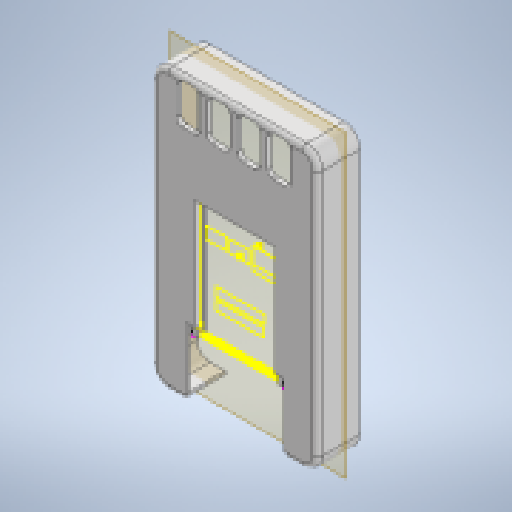
# Autodesk Inventor part: Top Housing
Saved by Autodesk Inventor 2023 (Build 270158000, 158)
## iProperties
Created: 2024-03-21
Part Number: Top Housing
Material: Generic
Document SubType Name: Modeling
Designer: Pobe Tran
Density: 1 g/cm^3
Appearance: Default
Author: Pobe Tran
Autodesk Inventor part; units mm, degrees
sketch "Sketch1" plane through (0, 0, 0) normal (0, 0, 1) x (1, 0, 0)
  point P0 (0, 0)
ref_plane "Work Plane1" through (48, 84.1076, 7.5) normal (0, 0, 1) x (1, 0, 0)
ref_plane "Work Plane2" through (-0.3396, -5.2087, 0) normal (0, 0, 1) x (1, 0, 0)
sketch "Sketch7" plane through (-0.3396, -5.2087, 0) normal (0, 0, 1) x (1, 0, 0)
  line L0 (50.1982, -77.6837) -> (50.1982, 77.6837) projected
  arc A0 (42.1982, -85.6837) -> (50.1982, -77.6837) centre (42.1982, -77.6837) ccw projected
  line L1 (-42.1982, -85.6837) -> (42.1982, -85.6837) projected
  line L2 (42.1982, -87.6837) -> (-42.1982, -87.6837) projected
  arc A1 (42.1982, -87.6837) -> (52.1982, -77.6837) centre (42.1982, -77.6837) ccw projected
  line L3 (52.1982, 77.6837) -> (52.1982, -77.6837) projected
  arc A2 (52.1982, 77.6837) -> (42.1982, 87.6837) centre (42.1982, 77.6837) ccw projected
  arc A3 (50.1982, 77.6837) -> (42.1982, 85.6837) centre (42.1982, 77.6837) ccw projected
  line L4 (-42.1982, 87.6837) -> (42.1982, 87.6837) projected
  line L5 (42.1982, 85.6837) -> (-42.1982, 85.6837) projected
  arc A4 (-42.1982, 87.6837) -> (-52.1982, 77.6837) centre (-42.1982, 77.6837) ccw projected
  arc A5 (-42.1982, 85.6837) -> (-50.1982, 77.6837) centre (-42.1982, 77.6837) ccw projected
  line L6 (-50.1982, 77.6837) -> (-50.1982, -77.6837) projected
  line L7 (-52.1982, -77.6837) -> (-52.1982, 77.6837) projected
  arc A6 (-52.1982, -77.6837) -> (-42.1982, -87.6837) centre (-42.1982, -77.6837) ccw projected
  arc A7 (-50.1982, -77.6837) -> (-42.1982, -85.6837) centre (-42.1982, -77.6837) ccw projected
  point P0 (0.3396, 5.2087)
extrude "Extrusion5" add sketch "Sketch7" along normal blind 11.5 and the other way blind 12
sketch "Sketch8" plane through (-0.3396, -5.2087, 11.5) normal (0, 0, 1) x (1, 0, 0)
  line L0 (52.1982, -77.6837) -> (52.1982, 77.6837) projected
  arc A0 (42.1982, -87.6837) -> (52.1982, -77.6837) centre (42.1982, -77.6837) ccw projected
  line L1 (-42.1982, -87.6837) -> (42.1982, -87.6837) projected
  arc A1 (-52.1982, -77.6837) -> (-42.1982, -87.6837) centre (-42.1982, -77.6837) ccw projected
  line L2 (-52.1982, 77.6837) -> (-52.1982, -77.6837) projected
  arc A2 (-42.1982, 87.6837) -> (-52.1982, 77.6837) centre (-42.1982, 77.6837) ccw projected
  line L3 (42.1982, 87.6837) -> (-42.1982, 87.6837) projected
  arc A3 (52.1982, 77.6837) -> (42.1982, 87.6837) centre (42.1982, 77.6837) ccw projected
  point P0 (0.3396, 5.2087)
extrude "Extrusion6" add sketch "Sketch8" along normal blind 3
sketch "Sketch9" plane through (-0.3396, -5.2087, 14.5) normal (0, 0, 1) x (1, 0, 0)
  arc A0 (31.6451, 60.9262) -> (34.8201, 64.1012) centre (31.6451, 64.1012) ccw projected
  line L0 (34.8201, 64.1012) -> (34.8201, 81.8812) projected
  arc A1 (34.8201, 81.8812) -> (31.6451, 85.0562) centre (31.6451, 81.8812) ccw projected
  line L1 (31.6451, 85.0562) -> (24.0251, 85.0562) projected
  arc A2 (24.0251, 85.0562) -> (20.8501, 81.8812) centre (24.0251, 81.8812) ccw projected
  line L2 (20.8501, 81.8812) -> (20.8501, 64.1012) projected
  arc A3 (20.8501, 64.1012) -> (24.0251, 60.9262) centre (24.0251, 64.1012) ccw projected
  line L3 (24.0251, 60.9262) -> (31.6451, 60.9262) projected
  arc A4 (12.5951, 60.9262) -> (15.7701, 64.1012) centre (12.5951, 64.1012) ccw projected
  line L4 (15.7701, 64.1012) -> (15.7701, 81.8812) projected
  arc A5 (15.7701, 81.8812) -> (12.5951, 85.0562) centre (12.5951, 81.8812) ccw projected
  line L5 (12.5951, 85.0562) -> (4.9751, 85.0562) projected
  arc A6 (4.9751, 85.0562) -> (1.8001, 81.8812) centre (4.9751, 81.8812) ccw projected
  line L6 (1.8001, 81.8812) -> (1.8001, 64.1012) projected
  arc A7 (1.8001, 64.1012) -> (4.9751, 60.9262) centre (4.9751, 64.1012) ccw projected
  line L7 (4.9751, 60.9262) -> (12.5951, 60.9262) projected
  arc A8 (-6.4549, 60.9262) -> (-3.2799, 64.1012) centre (-6.4549, 64.1012) ccw projected
  line L8 (-3.2799, 64.1012) -> (-3.2799, 81.8812) projected
  arc A9 (-3.2799, 81.8812) -> (-6.4549, 85.0562) centre (-6.4549, 81.8812) ccw projected
  line L9 (-6.4549, 85.0562) -> (-14.0749, 85.0562) projected
  arc A10 (-14.0749, 85.0562) -> (-17.2499, 81.8812) centre (-14.0749, 81.8812) ccw projected
  line L10 (-17.2499, 81.8812) -> (-17.2499, 64.1012) projected
  arc A11 (-17.2499, 64.1012) -> (-14.0749, 60.9262) centre (-14.0749, 64.1012) ccw projected
  line L11 (-14.0749, 60.9262) -> (-6.4549, 60.9262) projected
  arc A12 (-25.5049, 60.9262) -> (-22.3299, 64.1012) centre (-25.5049, 64.1012) ccw projected
  line L12 (-22.3299, 64.1012) -> (-22.3299, 81.8812) projected
  arc A13 (-22.3299, 81.8812) -> (-25.5049, 85.0562) centre (-25.5049, 81.8812) ccw projected
  line L13 (-25.5049, 85.0562) -> (-33.1249, 85.0562) projected
  arc A14 (-33.1249, 85.0562) -> (-36.2999, 81.8812) centre (-33.1249, 81.8812) ccw projected
  line L14 (-36.2999, 81.8812) -> (-36.2999, 64.1012) projected
  arc A15 (-36.2999, 64.1012) -> (-33.1249, 60.9262) centre (-33.1249, 64.1012) ccw projected
  line L15 (-33.1249, 60.9262) -> (-25.5049, 60.9262) projected
  arc A16 (31.6451, 60.4262) -> (35.3201, 64.1012) centre (31.6451, 64.1012) ccw
  line L16 (35.3201, 64.1012) -> (35.3201, 81.8812)
  arc A17 (35.3201, 81.8812) -> (31.6451, 85.5562) centre (31.6451, 81.8812) ccw
  line L17 (31.6451, 85.5562) -> (24.0251, 85.5562)
  arc A18 (24.0251, 85.5562) -> (20.3501, 81.8812) centre (24.0251, 81.8812) ccw
  line L18 (20.3501, 81.8812) -> (20.3501, 64.1012)
  arc A19 (20.3501, 64.1012) -> (24.0251, 60.4262) centre (24.0251, 64.1012) ccw
  line L19 (24.0251, 60.4262) -> (31.6451, 60.4262)
  line L20 (16.2701, 81.8812) -> (16.2701, 64.1012)
  arc A20 (12.5951, 60.4262) -> (16.2701, 64.1012) centre (12.5951, 64.1012) ccw
  line L21 (12.5951, 60.4262) -> (4.9751, 60.4262)
  arc A21 (1.3001, 64.1012) -> (4.9751, 60.4262) centre (4.9751, 64.1012) ccw
  line L22 (1.3001, 64.1012) -> (1.3001, 81.8812)
  arc A22 (4.9751, 85.5562) -> (1.3001, 81.8812) centre (4.9751, 81.8812) ccw
  line L23 (4.9751, 85.5562) -> (12.5951, 85.5562)
  arc A23 (16.2701, 81.8812) -> (12.5951, 85.5562) centre (12.5951, 81.8812) ccw
  arc A24 (-6.4549, 60.4262) -> (-2.7799, 64.1012) centre (-6.4549, 64.1012) ccw
  line L24 (-2.7799, 64.1012) -> (-2.7799, 81.8812)
  arc A25 (-2.7799, 81.8812) -> (-6.4549, 85.5562) centre (-6.4549, 81.8812) ccw
  line L25 (-6.4549, 85.5562) -> (-14.0749, 85.5562)
  arc A26 (-14.0749, 85.5562) -> (-17.7499, 81.8812) centre (-14.0749, 81.8812) ccw
  line L26 (-17.7499, 81.8812) -> (-17.7499, 64.1012)
  arc A27 (-17.7499, 64.1012) -> (-14.0749, 60.4262) centre (-14.0749, 64.1012) ccw
  line L27 (-14.0749, 60.4262) -> (-6.4549, 60.4262)
  arc A28 (-25.5049, 60.4262) -> (-21.8299, 64.1012) centre (-25.5049, 64.1012) ccw
  line L28 (-25.5049, 60.4262) -> (-33.1249, 60.4262)
  arc A29 (-36.7999, 64.1012) -> (-33.1249, 60.4262) centre (-33.1249, 64.1012) ccw
  line L29 (-36.7999, 64.1012) -> (-36.7999, 81.8812)
  arc A30 (-33.1249, 85.5562) -> (-36.7999, 81.8812) centre (-33.1249, 81.8812) ccw
  line L30 (-33.1249, 85.5562) -> (-25.5049, 85.5562)
  arc A31 (-21.8299, 81.8812) -> (-25.5049, 85.5562) centre (-25.5049, 81.8812) ccw
  line L31 (-21.8299, 81.8812) -> (-21.8299, 64.1012)
  point P0 (0.3396, 5.2087)
  dimension "d28" = 0.5
  dimension "d29" = 0.5
  dimension "d30" = 0.5
  dimension "d31" = 0.5
  constraints: 32 end point, 32 point on circle, 16 centre point, 28 other
  measures "d28" distance between parallel lines of L3 L19
  measures "d29" distance between parallel lines of L4 L20
  measures "d30" distance between parallel lines of L11 L27
  measures "d31" radial gap between concentric circles of A12 A28
extrude "Extrusion7" cut sketch "Sketch9" against normal blind 3 contours L3 A3 L2 A2 L1 A1 L0 A0 | L7 A7 L6 A6 L5 A5 L4 A4 | L11 A11 L10 A10 L9 A9 L8 A8 | L15 A15 L14 A14 L13 A13 L12 A12 | L19 A19 L18 A18 L17 A17 L16 A16 | L20 A20 L21 A21 L22 A22 L23 A23 | L27 A27 L26 A26 L25 A25 L24 A24 | L28 A29 L29 A30 L30 A31 L31 A28
sketch "Sketch10" plane through (-0.3396, -5.2087, 14.5) normal (0, 0, 1) x (1, 0, 0)
  line L0 (25.0411, 23.7903) -> (-24.5651, 23.7903) projected
  line L1 (-24.5651, 23.7903) -> (-24.5651, -45.0437) projected
  line L2 (-24.5651, -45.0437) -> (25.0411, -45.0437) projected
  line L3 (25.0411, -45.0437) -> (25.0411, 23.7903) projected
  line L4 (-28.4005, 30.4451) -> (28.6225, 30.4451) projected
  line L5 (28.6225, -51.2159) -> (-28.4005, -51.2159) projected
  line L6 (-25.2255, -45.5009) -> (-25.2255, 24.7301) projected
  line L7 (25.5411, 24.2903) -> (-25.0651, 24.2903)
  line L8 (-25.0651, 24.2903) -> (-25.0651, -45.5437)
  line L9 (-25.0651, -45.5437) -> (25.5411, -45.5437)
  line L10 (25.5411, -45.5437) -> (25.5411, 24.2903)
  dimension "d34" = 0.5
  constraints: 8 end point, 3 other
  measures "d34" distance between parallel lines of L3 L10
extrude "Extrusion8" cut sketch "Sketch10" against normal blind 3 contours L3 L2 L1 L0 | L10 L9 L8 L7
fillet "Fillet1" radius 3.175 8 edges at (48.9297, 79.546, 14.5) (-0.3396, 82.475, 14.5) (-49.609, 79.546, 14.5) (-52.5379, -5.2087, 14.5) (-49.609, -89.9635, 14.5) (-0.3396, -92.8924, 14.5) (48.9297, -89.9635, 14.5) (51.8586, -5.2087, 14.5)
sketch "Sketch15" plane through (-0.3396, -5.2087, 11.5) normal (0, 0, -1) x (-1, 0, 0)
  line L0 (-28.6225, -51.2159) -> (28.4005, -51.2159) projected
  arc A0 (28.4005, -51.2159) -> (28.4005, -46.0089) centre (28.4005, -48.6124) ccw projected
  line L1 (28.4005, -46.0089) -> (25.7335, -46.0089) projected
  arc A1 (25.2255, -45.5009) -> (25.7335, -46.0089) centre (25.7335, -45.5009) ccw projected
  line L2 (25.2255, -45.5009) -> (25.2255, 24.7301) projected
  arc A2 (25.7335, 25.2381) -> (25.2255, 24.7301) centre (25.7335, 24.7301) ccw projected
  line L3 (25.7335, 25.2381) -> (28.4005, 25.2381) projected
  arc A3 (28.4005, 25.2381) -> (28.4005, 30.4451) centre (28.4005, 27.8416) ccw projected
  line L4 (28.4005, 30.4451) -> (-28.6225, 30.4451) projected
  arc A4 (-28.6225, 30.4451) -> (-28.6225, 25.2381) centre (-28.6225, 27.8416) ccw projected
  line L5 (-28.6225, 25.2381) -> (-25.9555, 25.2381) projected
  arc A5 (-25.4475, 24.7301) -> (-25.9555, 25.2381) centre (-25.9555, 24.7301) ccw projected
  line L6 (-25.4475, 24.7301) -> (-25.4475, -45.5009) projected
  arc A6 (-25.9555, -46.0089) -> (-25.4475, -45.5009) centre (-25.9555, -45.5009) ccw projected
  line L7 (-25.9555, -46.0089) -> (-28.6225, -46.0089) projected
  arc A7 (-28.6225, -46.0089) -> (-28.6225, -51.2159) centre (-28.6225, -48.6124) ccw projected
  circle A8 centre (-18.6861, 27.9216) radius 0.9995 projected
  circle A9 centre (-16.1861, 27.9216) radius 0.9995 projected
  circle A10 centre (-13.6861, 27.9216) radius 0.9995 projected
  circle A11 centre (-11.1861, 27.9216) radius 0.9995 projected
  circle A12 centre (-8.6861, 27.9216) radius 0.9995 projected
  circle A13 centre (-6.1861, 27.9216) radius 0.9995 projected
  circle A14 centre (-3.6861, 27.9216) radius 0.9995 projected
  circle A15 centre (-1.1861, 27.9216) radius 0.9995 projected
  circle A16 centre (1.3139, 27.9216) radius 0.9995 projected
  circle A17 centre (3.8139, 27.9216) radius 0.9995 projected
  circle A18 centre (6.3139, 27.9216) radius 0.9995 projected
  circle A19 centre (8.8139, 27.9216) radius 0.9995 projected
  circle A20 centre (11.3139, 27.9216) radius 0.9995 projected
  circle A21 centre (13.8139, 27.9216) radius 0.9995 projected
  circle A22 centre (16.3139, 27.9216) radius 0.9995 projected
  circle A23 centre (18.8139, 27.9216) radius 0.9995 projected
  circle A24 centre (21.3139, 27.9216) radius 0.9995 projected
  line L8 (24.8139, -49.6924) -> (24.8139, -47.6924) projected
  line L9 (22.8139, -49.6924) -> (24.8139, -49.6924) projected
  line L10 (22.8139, -47.6924) -> (22.8139, -49.6924) projected
  line L11 (24.8139, -47.6924) -> (22.8139, -47.6924) projected
  line L12 (21.5552, 3.8513) -> (21.5552, 11.3443) projected
  line L13 (8.6012, 3.8513) -> (21.5552, 3.8513) projected
  line L14 (8.6012, 11.3443) -> (8.6012, 3.8513) projected
  line L15 (21.5552, 11.3443) -> (8.6012, 11.3443) projected
  line L16 (6.5692, 3.8513) -> (6.5692, 11.3443) projected
  line L17 (-6.3848, 3.8513) -> (6.5692, 3.8513) projected
  line L18 (-6.3848, 11.3443) -> (-6.3848, 3.8513) projected
  line L19 (6.5692, 11.3443) -> (-6.3848, 11.3443) projected
  line L20 (15.3703, -24.4189) -> (15.3703, -18.9325) projected
  line L21 (-15.1097, -24.4189) -> (15.3703, -24.4189) projected
  line L22 (-15.1097, -18.9325) -> (-15.1097, -24.4189) projected
  line L23 (15.3703, -18.9325) -> (-15.1097, -18.9325) projected
  line L24 (-14.9827, -31.7849) -> (15.0147, -31.7849) projected
  line L25 (-14.9827, -26.2858) -> (-14.9827, -31.7849) projected
  line L26 (15.0147, -26.2858) -> (-14.9827, -26.2858) projected
  line L27 (15.0147, -31.7849) -> (15.0147, -26.2858) projected
  arc A25 (-22.359, 3.3941) -> (-21.8579, 4.9181) centre (-36.9264, 9.0284) ccw projected
  line L28 (-8.0739, 4.9181) -> (-21.8579, 4.9181) projected
  line L29 (-8.0739, 4.9181) -> (-8.0739, 14.9003) projected
  line L30 (-8.0739, 14.9003) -> (-22.4531, 14.9003) projected
  arc A26 (-22.4531, 14.9003) -> (-22.5265, 15.0781) centre (-36.9264, 9.0284) ccw projected
  line L31 (-7.8961, 15.0781) -> (-22.5265, 15.0781) projected
  line L32 (-7.8961, 1.1081) -> (-7.8961, 15.0781) projected
  line L33 (-23.1615, 1.1081) -> (-7.8961, 1.1081) projected
  line L34 (-23.1615, 3.3941) -> (-23.1615, 1.1081) projected
  line L35 (-22.359, 3.3941) -> (-23.1615, 3.3941) projected
  arc A27 (-24.6855, -48.6886) -> (-22.6866, -48.6886) centre (-23.6861, -48.6924) ccw projected
  arc A28 (-22.6866, -48.6886) -> (-24.6855, -48.6886) centre (-23.6861, -48.6848) ccw projected
  arc A29 (-22.1855, -48.6886) -> (-20.1866, -48.6886) centre (-21.1861, -48.6924) ccw projected
  arc A30 (-20.1866, -48.6886) -> (-22.1855, -48.6886) centre (-21.1861, -48.6848) ccw projected
  arc A31 (-19.6855, -48.6886) -> (-17.6866, -48.6886) centre (-18.6861, -48.6924) ccw projected
  arc A32 (-17.6866, -48.6886) -> (-19.6855, -48.6886) centre (-18.6861, -48.6848) ccw projected
  arc A33 (-17.1855, -48.6886) -> (-15.1866, -48.6886) centre (-16.1861, -48.6924) ccw projected
  arc A34 (-15.1866, -48.6886) -> (-17.1855, -48.6886) centre (-16.1861, -48.6848) ccw projected
  arc A35 (-14.6855, -48.6886) -> (-12.6866, -48.6886) centre (-13.6861, -48.6924) ccw projected
  arc A36 (-12.6866, -48.6886) -> (-14.6855, -48.6886) centre (-13.6861, -48.6848) ccw projected
  arc A37 (-12.1855, -48.6886) -> (-10.1866, -48.6886) centre (-11.1861, -48.6924) ccw projected
  arc A38 (-10.1866, -48.6886) -> (-12.1855, -48.6886) centre (-11.1861, -48.6848) ccw projected
  arc A39 (-9.6855, -48.6886) -> (-7.6866, -48.6886) centre (-8.6861, -48.6924) ccw projected
  arc A40 (-7.6866, -48.6886) -> (-9.6855, -48.6886) centre (-8.6861, -48.6848) ccw projected
  arc A41 (-7.1855, -48.6886) -> (-5.1866, -48.6886) centre (-6.1861, -48.6924) ccw projected
  arc A42 (-5.1866, -48.6886) -> (-7.1855, -48.6886) centre (-6.1861, -48.6848) ccw projected
  arc A43 (-4.6855, -48.6886) -> (-2.6866, -48.6886) centre (-3.6861, -48.6924) ccw projected
  arc A44 (-2.6866, -48.6886) -> (-4.6855, -48.6886) centre (-3.6861, -48.6848) ccw projected
  arc A45 (-2.1855, -48.6886) -> (-0.1866, -48.6886) centre (-1.1861, -48.6924) ccw projected
  arc A46 (-0.1866, -48.6886) -> (-2.1855, -48.6886) centre (-1.1861, -48.6848) ccw projected
  arc A47 (0.3145, -48.6886) -> (2.3134, -48.6886) centre (1.3139, -48.6924) ccw projected
  arc A48 (2.3134, -48.6886) -> (0.3145, -48.6886) centre (1.3139, -48.6848) ccw projected
  arc A49 (2.8145, -48.6886) -> (4.8134, -48.6886) centre (3.8139, -48.6924) ccw projected
  arc A50 (4.8134, -48.6886) -> (2.8145, -48.6886) centre (3.8139, -48.6848) ccw projected
  arc A51 (5.3145, -48.6886) -> (7.3134, -48.6886) centre (6.3139, -48.6924) ccw projected
  arc A52 (7.3134, -48.6886) -> (5.3145, -48.6886) centre (6.3139, -48.6848) ccw projected
  arc A53 (7.8145, -48.6886) -> (9.8134, -48.6886) centre (8.8139, -48.6924) ccw projected
  arc A54 (9.8134, -48.6886) -> (7.8145, -48.6886) centre (8.8139, -48.6848) ccw projected
  arc A55 (10.3145, -48.6886) -> (12.3134, -48.6886) centre (11.3139, -48.6924) ccw projected
  arc A56 (12.3134, -48.6886) -> (10.3145, -48.6886) centre (11.3139, -48.6848) ccw projected
  arc A57 (12.8145, -48.6886) -> (14.8134, -48.6886) centre (13.8139, -48.6924) ccw projected
  arc A58 (14.8134, -48.6886) -> (12.8145, -48.6886) centre (13.8139, -48.6848) ccw projected
  arc A59 (15.3145, -48.6886) -> (17.3134, -48.6886) centre (16.3139, -48.6924) ccw projected
  arc A60 (17.3134, -48.6886) -> (15.3145, -48.6886) centre (16.3139, -48.6848) ccw projected
  arc A61 (17.8145, -48.6886) -> (19.8134, -48.6886) centre (18.8139, -48.6924) ccw projected
  arc A62 (19.8134, -48.6886) -> (17.8145, -48.6886) centre (18.8139, -48.6848) ccw projected
  arc A63 (20.3145, -48.6886) -> (22.3134, -48.6886) centre (21.3139, -48.6924) ccw projected
  arc A64 (22.3134, -48.6886) -> (20.3145, -48.6886) centre (21.3139, -48.6848) ccw projected
  line L36 (22.8139, 28.9216) -> (24.8139, 28.9216) projected
  line L37 (24.8139, 28.9216) -> (24.8139, 26.9216) projected
  line L38 (24.8139, 26.9216) -> (22.8139, 26.9216) projected
  line L39 (22.8139, 26.9216) -> (22.8139, 28.9216) projected
  circle A65 centre (-21.1861, 27.9216) radius 0.9995 projected
  circle A66 centre (-23.6861, 27.9216) radius 0.9995 projected
  circle A67 centre (28.4005, 27.8416) radius 2.032 projected
  circle A68 centre (28.4005, -48.6124) radius 2.032 projected
  circle A69 centre (-28.6225, -48.6124) radius 2.032 projected
  circle A70 centre (-28.6225, 27.8416) radius 2.032 projected
  arc A71 (31.004, 27.8416) -> (25.797, 27.8416) centre (28.4005, 27.8416) ccw
  line L40 (28.4005, -51.2159) -> (-28.6225, -51.2159) projected
  arc A72 (25.797, -48.6124) -> (31.004, -48.6124) centre (28.4005, -48.6124) ccw
  line L41 (31.004, 27.8416) -> (31.004, -48.6124)
  line L42 (25.797, 27.8416) -> (25.797, -48.6124)
  arc A73 (-26.019, 27.8416) -> (-31.226, 27.8416) centre (-28.6225, 27.8416) ccw
  arc A74 (-31.226, -48.6124) -> (-26.019, -48.6124) centre (-28.6225, -48.6124) ccw
  line L43 (-31.226, 27.8416) -> (-31.226, -48.6124)
  line L44 (-26.019, 27.8416) -> (-26.019, -48.6124)
  point P0 (-0.3396, 5.2087)
  point P1 (28.4005, 30.4451)
  point P2 (-28.6225, 30.4451)
  point P3 (-28.6225, -51.2159)
  constraints: 13 point on circle, 12 end point, 4 centre point, 4 coincident, 2 tangent, 1 concentric
sketch "Sketch17" plane through (-0.3396, -5.2087, 11.5) normal (0, 0, -1) x (-1, 0, 0)
  line L0 (-31.226, 27.8416) -> (-31.226, -48.6124) projected
  line L1 (31.004, -48.6124) -> (31.004, 27.8416) projected
  arc A0 (-28.6225, -46.0089) -> (-28.6225, -51.2159) centre (-28.6225, -48.6124) ccw construction
  line L2 (-25.5411, -45.5437) -> (25.0651, -45.5437) projected
  line L3 (-25.5411, -45.5437) -> (25.0651, -45.5437)
  line L4 (25.0651, -45.5437) -> (25.0651, -51.2159)
  line L5 (25.0651, -51.2159) -> (-25.5411, -51.2159)
  line L6 (-25.5411, -51.2159) -> (-25.5411, -45.5437)
  line L7 (25.0651, 24.2903) -> (-25.5411, 24.2903) projected
  line L8 (-25.5411, 24.2903) -> (25.0651, 24.2903)
  line L9 (25.0651, 24.2903) -> (25.0651, 30.4359)
  line L10 (25.0651, 30.4359) -> (-25.5411, 30.4359)
  line L11 (-25.5411, 30.4359) -> (-25.5411, 24.2903)
  point P0 (-0.3396, 5.2087)
  point P1 (25.0651, -45.5437)
  constraints: 16 end point, 4 parallel, 2 horizontal, 2 perpendicular, 1 point on line
extrude "Extrusion14" cut sketch "Sketch17" against normal blind 1.5
sketch "Sketch18" plane through (-0.3396, -5.2087, 11.5) normal (0, 0, -1) x (-1, 0, 0)
  line L0 (-31.226, 27.8416) -> (-31.226, -48.6124) projected
  line L1 (31.004, -48.6124) -> (31.004, 27.8416) projected
  arc A0 (31.004, 27.8416) -> (25.797, 27.8416) centre (28.4005, 27.8416) ccw projected
  arc A1 (-26.019, 27.8416) -> (-31.226, 27.8416) centre (-28.6225, 27.8416) ccw projected
  line L2 (-32.926, -48.6124) -> (-32.926, 32.1451)
  line L3 (32.704, -48.6124) -> (32.704, 27.8416)
  line L4 (-31.426, -48.6124) -> (-31.426, 27.8416)
  arc A2 (-25.819, 27.8416) -> (-31.426, 27.8416) centre (-28.6225, 27.8416) ccw
  line L5 (31.204, -48.6124) -> (31.204, 27.8416)
  arc A3 (31.204, 27.8416) -> (25.598, 27.9178) centre (28.4005, 27.8416) ccw
  line L6 (32.704, 32.1449) -> (32.704, 27.8416)
  line L7 (31.204, 27.8416) -> (31.204, 30.6449)
  line L8 (-31.426, 27.8416) -> (-31.426, 30.6451)
  line L9 (-25.5411, 30.4359) -> (25.0651, 30.4359) projected
  line L10 (-25.5411, 30.4359) -> (-24.0411, 30.4359) construction
  line L11 (-25.5411, 32.1451) -> (-32.926, 32.1451)
  line L12 (-31.426, 30.6451) -> (-25.5411, 30.6451)
  line L13 (-25.5411, 32.1451) -> (-25.5411, 30.6451)
  line L14 (31.204, 30.6449) -> (25.0651, 30.6449)
  line L15 (25.0651, 30.6449) -> (25.0651, 32.1449)
  line L16 (25.0651, 32.1449) -> (32.704, 32.1449)
  line L17 (-25.5411, 32.1451) -> (-32.9222, 32.1451)
  line L18 (-32.9222, 32.1451) -> (-32.9222, -51.2159)
  line L19 (-32.9222, -51.2159) -> (-25.5411, -51.2159)
  line L20 (-25.5411, -51.2159) -> (-25.5411, 32.1451)
  line L21 (25.0651, -51.2159) -> (-25.5411, -51.2159) projected
  line L22 (25.0651, 30.4359) -> (25.0651, -51.2159) projected
  line L23 (25.0651, -51.2159) -> (32.704, -51.2159)
  line L24 (32.704, -51.2159) -> (32.704, 32.1449)
  line L25 (32.704, 32.1449) -> (25.0651, 32.1449)
  line L26 (25.0651, 32.1449) -> (25.0651, -51.2159)
  point P0 (-0.3396, 5.2087)
  point P1 (25.0651, 30.4359)
  dimension "d66" = 1.7
  dimension "d67" = 1.7
  dimension "d68" = 0.2
  dimension "d69" = 0.2
  dimension "d72" = 1.5
  dimension "d73" = 1.5
  constraints: 44 end point, 5 horizontal, 4 parallel, 4 perpendicular, 4 point on circle, 3 vertical, 2 centre point, 1 point on line, 1 tangent, 2 other
  measures "d66" distance between parallel lines of L0 L2
  measures "d67" distance between parallel lines of L1 L3
  measures "d68" distance between parallel lines of L0 L4
  measures "d69" distance between parallel lines of L1 L5
  measures "d72" distance between parallel lines of L11 L12
  measures "d73" distance of L14.end L15.end
extrude "Extrusion16" add sketch "Sketch18" along normal blind 4.5 contours L24 L23 L22 L26 L15 L16 L6 L3 | L19 L18 L11 L13 L20 | A2 L8 L12 | A3 L14 L7
sketch "Sketch20" plane through (-42.5379, -92.8924, -12) normal (0, -1, 0) x (1, 0, 0)
  line L0 (9.4943, 23.5) -> (9.4943, 19) projected
  line L1 (75.1204, 23.5) -> (75.1204, 19) projected
  line L2 (84.3965, 26.5) -> (0, 26.5) projected
  line L3 (0, 0) -> (84.3965, 0) projected
  line L4 (9.4943, 26.5) -> (75.1204, 26.5)
  line L5 (75.1204, 26.5) -> (75.1204, 0)
  line L6 (75.1204, 0) -> (9.4943, 0)
  line L7 (9.4943, 0) -> (9.4943, 26.5)
  point P0 (17.1332, 26.5)
  point P1 (9.4943, 0)
  point P2 (75.1204, 26.5)
  constraints: 8 end point, 2 parallel, 2 point on line, 1 horizontal, 1 perpendicular
extrude "Extrusion19" cut sketch "Sketch20" against normal up to surface (36.4678 mm away)
sketch "Sketch23" plane through (-25.4047, -56.4246, 13) normal (0, -1, 0) x (1, 0, 0)
  line L0 (0, 1.5) -> (0, 0) projected
  line L1 (50.6062, 1.5) -> (50.6062, 0) projected
  line L2 (0, 1.5) -> (50.6062, 1.5)
  line L3 (50.6062, 1.5) -> (50.6062, 0)
  line L4 (50.6062, 0) -> (0, 0)
  line L5 (0, 0) -> (0, 1.5)
  point P0 (25.4047, -13)
  constraints: 8 end point, 2 parallel, 1 horizontal, 1 perpendicular
ref_plane "Work Plane3" through (-24.9047, 18.5816, 12.9384) normal (0, 1, 0) x (0, 0, 1)
extrude "Extrusion20" cut sketch "Sketch23" against normal up to surface (75.0062 mm away)
sketch "Sketch24" plane through (-33.0436, -56.4246, 7) normal (0, -1, 0) x (1, 0, 0)
  line L0 (0, 7.5) -> (7.6389, 7.5) projected
  line L1 (0, 7.5) -> (2, 7.5)
  line L2 (2, 7.5) -> (2, 5.8)
  line L3 (2, 5.8) -> (0, 5.8)
  line L4 (0, 5.8) -> (0, 7.5)
  line L5 (74.9022, 7.5) -> (65.6261, 7.5) projected
  line L6 (65.6261, 7.5) -> (63.6261, 7.5)
  line L7 (63.6261, 7.5) -> (63.6261, 5.8)
  line L8 (63.6261, 5.8) -> (65.6261, 5.8)
  line L9 (65.6261, 5.8) -> (65.6261, 7.5)
  point P0 (33.0436, -7)
  point P1 (2, 7.5)
  dimension "d87" = 2
  dimension "d88" = 1.7
  dimension "d89" = 2
  constraints: 16 end point, 4 parallel, 2 horizontal, 2 perpendicular, 1 point on line
  measures "d87" distance of L2.end L3.end
  measures "d88" distance of L1.end L2.end
  measures "d89" distance of L8.end L7.end
extrude "Extrusion21" add sketch "Sketch24" along normal up to surface (33.2928 mm away)
sketch "Sketch25" plane through (-33.0436, -56.4246, 7) normal (0, -1, 0) x (1, 0, 0)
  line L0 (2, 7.5) -> (2, 5.8) projected
  line L1 (63.6261, 5.8) -> (63.6261, 7.5) projected
  line L2 (2, 7.5) -> (63.6261, 7.5)
  line L3 (63.6261, 7.5) -> (63.6261, 5.8)
  line L4 (63.6261, 5.8) -> (2, 5.8)
  line L5 (2, 5.8) -> (2, 7.5)
  point P0 (33.0436, -7)
  point P1 (2, 5.8)
  constraints: 8 end point, 2 parallel, 1 horizontal, 1 perpendicular
ref_plane "Work Plane4" through (-24.9047, -50.2524, 12.9384) normal (0, -1, 0) x (1, 0, 0)
extrude "Extrusion22" cut sketch "Sketch25" against normal up to surface (6.1722 mm away)
sketch "Sketch27" plane through (-33.0436, -56.4246, 7) normal (0, -1, 0) x (1, 0, 0)
  line L0 (1.7, 4.5) -> (4.3035, 4.5) projected
  line L1 (61.3265, 4.5) -> (63.93, 4.5) projected
  line L2 (61.3265, 1.476) -> (4.3035, 1.476)
  line L3 (1.7, 4.5) -> (63.93, 4.5)
  line L4 (63.93, 4.5) -> (63.93, 2.226)
  line L5 (63.93, 2.226) -> (1.7, 2.226)
  line L6 (1.7, 2.226) -> (1.7, 4.5)
  line L7 (1.4, 4.8) -> (64.23, 4.8)
  line L8 (64.23, 4.8) -> (64.23, 1.926)
  line L9 (64.23, 1.926) -> (1.4, 1.926)
  line L10 (1.4, 1.926) -> (1.4, 4.8)
  point P0 (33.0436, -7)
  point P1 (4.3035, 4.5)
  point P2 (61.3265, 4.5)
  dimension "d98" = 62.23
  dimension "d99" = 0.3
  constraints: 18 end point, 4 parallel, 2 horizontal, 2 perpendicular, 5 other
  measures "d98" distance between parallel lines of L4 L6
  measures "d99" distance between parallel lines of L6 L10
extrude "Extrusion24" cut sketch "Sketch27" against normal blind 82.1 contours L0 L3 L1 L4 L5 L6 | L7 L8 L9 L10
move faces "Move1" translate (-0.75, 0, 0) faces at (-33.0436, -0.8508, 10)
move faces "Move2" translate (0.75, 0, 0) faces at (32.5825, -0.8506, 10)
move faces "Move4" translate (0, 0, -0.5) faces at (-29.564, -1.8407, 11.8)
sketch "Sketch28" plane through (-52.5379, -82.8924, -12) normal (-1, 0, 0) x (0, 0, 1)
  arc A0 (0, 93.5902) -> (0, 87.6638) centre (2, 90.627) ccw
  circle A1 centre (2, 90.627) radius 3.575 projected
  point P0 (12, 82.8924)
  constraints: 2 point on circle, 1 centre point, 4 other
extrude "Extrusion25" cut sketch "Sketch28" against normal blind 3
body "Solid2"
